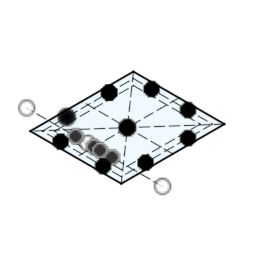
FrontPanelSwitchesLeds v3 (Autodesk Fusion 360 design; units mm, degrees)
Autodesk Fusion 360 part; units mm, degrees
sketch "Sketch1" plane through (0, 0, 0) normal (0, 0, 1) x (-1, 0, 0)
  line L0 (75, -85) -> (-75, -85)
  line L1 (-75, -85) -> (-75, 85)
  line L2 (-75, 85) -> (75, 85)
  line L3 (75, 85) -> (75, -85)
  line L4 (75, -85) -> (-75, 85) construction
  line L5 (-75, -85) -> (75, 85) construction
  line L6 (-55, 65) -> (55, 65) construction
  line L7 (55, 65) -> (55, -65) construction
  line L8 (55, -65) -> (-55, -65) construction
  line L9 (-55, -65) -> (-55, 65) construction
  line L10 (-65, 75) -> (65, 75) construction
  line L11 (65, 75) -> (65, -75) construction
  line L12 (65, -75) -> (-65, -75) construction
  line L13 (-65, -75) -> (-65, 75) construction
  line L14 (-112.9444, 55) -> (110.8284, 55) construction
  line L15 (30.2645, 52.25) -> (-29.7355, 52.25) construction
  line L16 (-29.7355, 52.25) -> (-29.7355, 57.75) construction
  line L17 (-29.7355, 57.75) -> (30.2645, 57.75) construction
  line L18 (30.2645, 57.75) -> (30.2645, 52.25) construction
  line L19 (30.2645, 52.25) -> (-29.7355, 57.75) construction
  line L20 (-29.7355, 52.25) -> (30.2645, 57.75) construction
  line L21 (-29.7355, 57.75) -> (-9.7355, 57.75) construction
  line L22 (-9.7355, 57.75) -> (-9.7355, 52.25) construction
  line L23 (-9.7355, 52.25) -> (-29.7355, 52.25) construction
  line L24 (-29.7355, 52.25) -> (-29.7355, 57.75) construction
  line L25 (-9.7355, 57.75) -> (10.2645, 57.75) construction
  line L26 (10.2645, 57.75) -> (10.2645, 52.25) construction
  line L27 (10.2645, 52.25) -> (-9.7355, 52.25) construction
  line L28 (-9.7355, 52.25) -> (-9.7355, 57.75) construction
  line L29 (-25.4805, 50.795) -> (-33.9905, 50.795)
  line L30 (-33.9905, 50.795) -> (-33.9905, 59.205)
  line L31 (-33.9905, 59.205) -> (-25.4805, 59.205)
  line L32 (-25.4805, 59.205) -> (-25.4805, 50.795)
  line L33 (-25.4805, 50.795) -> (-33.9905, 59.205) construction
  line L34 (-33.9905, 50.795) -> (-25.4805, 59.205) construction
  line L35 (34.5195, 50.795) -> (26.0095, 50.795)
  line L36 (26.0095, 50.795) -> (26.0095, 59.205)
  line L37 (26.0095, 59.205) -> (34.5195, 59.205)
  line L38 (34.5195, 59.205) -> (34.5195, 50.795)
  line L39 (34.5195, 50.795) -> (26.0095, 59.205) construction
  line L40 (26.0095, 50.795) -> (34.5195, 59.205) construction
  circle A0 centre (-9.7355, 55) radius 2.5
  line L41 (-9.7355, 57.75) -> (0.2645, 57.75) construction
  line L42 (0.2645, 57.75) -> (0.2645, 52.25) construction
  line L43 (0.2645, 52.25) -> (-9.7355, 52.25) construction
  line L44 (-9.7355, 52.25) -> (-9.7355, 57.75) construction
  circle A1 centre (10.2645, 55) radius 2.5
  circle A2 centre (-65, -35) radius 2.55
  circle A3 centre (-65, 35) radius 2.55
  line L45 (0, -85) -> (0, 85) construction
  line L46 (-75, 0) -> (75, 0) construction
  circle A4 centre (65, 35) radius 2.55
  circle A5 centre (65, -35) radius 2.55
  circle A6 centre (65, 35) radius 2.55
  circle A7 centre (-25, -75) radius 2.55
  circle A8 centre (35, -75) radius 2.55
  circle A9 centre (-35, 75) radius 2.55
  circle A10 centre (35, 75) radius 2.55
  point P0 (0.2645, 55)
  point P1 (-29.7355, 55)
  point P2 (30.2645, 55)
  point P3 (65, -35)
  dimension "d1" = 150
  dimension "d2" = 170
  dimension "d3" = 20
  dimension "d4" = 10
  dimension "d5" = 10
  dimension "d6" = 60
  dimension "d7" = 5.5
  dimension "d8" = 20
  dimension "d9" = 20
  dimension "d10" = 8.51
  dimension "d11" = 8.41
  dimension "d12" = 8.51
  dimension "d13" = 8.41
  dimension "d14" = 5
  dimension "d16" = 5.1
  dimension "d17" = 40
  dimension "d18" = 5.1
  dimension "d19" = 70
  dimension "d20" = 5.1
  dimension "d21" = 5.1
  dimension "d22" = 5.1
  dimension "d23" = 5.1
  dimension "d24" = 40
  dimension "d25" = 40
  dimension "d26" = 5.1
  dimension "d27" = 5.1
  dimension "d28" = 40
  dimension "d29" = 40
  constraint horizontal L0
  constraint perpendicular L0 L1
  constraint parallel L0 L2
  constraint parallel L1 L3
  constraint coincident L4 origin
  constraint coincident L5 origin
  constraint perpendicular L3 L14
  constraint horizontal L15
  constraint perpendicular L15 L16
  constraint parallel L15 L17
  constraint parallel L16 L18
  constraint coincident L19 P0
  constraint coincident L20 P0
  constraint coincident L14 P0
  constraint horizontal L21
  constraint vertical L22
  constraint horizontal L23
  constraint vertical L24
  constraint horizontal L25
  constraint vertical L26
  constraint horizontal L27
  constraint vertical L28
  constraint horizontal L29
  constraint perpendicular L29 L30
  constraint parallel L29 L31
  constraint parallel L30 L32
  constraint coincident L33 P1
  constraint coincident L34 P1
  constraint midpoint L16 P1
  constraint horizontal L35
  constraint perpendicular L35 L36
  constraint parallel L35 L37
  constraint parallel L36 L38
  constraint coincident L39 P2
  constraint coincident L40 P2
  constraint midpoint L18 P2
  constraint midpoint L22 A0.centre
  constraint horizontal L41
  constraint vertical L42
  constraint horizontal L43
  constraint vertical L44
  constraint midpoint L15 L42.end
  constraint symmetric A0 L42 A1
  constraint coincident L13 A2.centre
  constraint coincident L13 A3.centre
  constraint midpoint L0 L45.start
  constraint midpoint L2 L45.end
  constraint midpoint L1 L46.start
  constraint midpoint L3 L46.end
  constraint symmetric A2.centre L45 P3
  constraint symmetric A3 L45 A4
  constraint coincident P3 A5.centre
  constraint concentric A4 A6
  constraint coincident L12 A7.centre
  constraint coincident L12 A8.centre
  constraint coincident L10 A9.centre
  constraint coincident L10 A10.centre
  measures "d1" distance of L1.end L2.end
  measures "d2" distance of L0.end L1.end
  measures "d5" distance of L6 L14
  measures "d6" distance of L16.end L17.end
  measures "d7" distance of L15.end L16.end
  measures "d8" distance of L16.end L21.end
  measures "d9" distance of L21.end L25.end
  measures "d10" distance of L30.end L31.end
  measures "d11" distance of L29.end L30.end
  measures "d12" distance of L36.end L37.end
  measures "d13" distance of L35.end L36.end
  measures "d14" diameter of A0
  measures "d16" diameter of A2
  measures "d17" distance of L12 A2.centre
  measures "d18" diameter of A3
  measures "d19" distance of A2.centre A3.centre
  measures "d20" diameter of A5
  measures "d21" diameter of A6
  measures "d22" diameter of A7
  measures "d23" diameter of A8
  measures "d24" distance of L13 A7.centre
  measures "d25" distance of L3 A8.centre
  measures "d26" diameter of A9
  measures "d27" diameter of A10
  measures "d28" distance of L1 A9.centre
  measures "d29" distance of L3 A10.centre
extrude "Extrude1" add sketch "Sketch1" along normal blind 6 contours L0 L1 L2 L3 | A0 | A1 makes body 1
ref_plane "WorkPlane1" through (0, 0, 6) normal (0, 0, 1) x (-1, 0, 0)
extrude "Extrude2" add sketch "Sketch1" along normal blind 6 separate body makes body 2
hidden bodies 2
